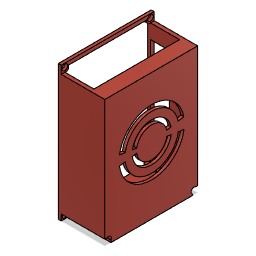
крышка на расбери v2 (Autodesk Fusion 360 design; units mm, degrees)
Autodesk Fusion 360 part; units mm, degrees
sketch "Sketch1" plane through (0, 0, 0) normal (1, 0, 0) x (0, 1, 0)
  line L0 (-75, 50) -> (13, 50)
  line L1 (13, 50) -> (13, -9)
  line L2 (13, -9) -> (-75, -9)
  line L3 (-75, -9) -> (-75, 50)
  circle A0 centre (-75, 50) radius 2
  circle A1 centre (13, 50) radius 2
  circle A2 centre (-75, -9) radius 2
  circle A3 centre (13, -9) radius 2
  line L4 (-77.5, 52.5) -> (-77.5, 47.5)
  line L5 (-77.5, 47.5) -> (-74, 47.5)
  line L6 (-72.5, 49) -> (-72.5, 52.5)
  line L7 (-72.5, 52.5) -> (10, 52.5)
  line L8 (10, 52.5) -> (10, 49)
  line L9 (11.5, 47.5) -> (15.5, 47.5)
  line L10 (15.5, 47.5) -> (15.5, 52.5)
  line L11 (15.5, 52.5) -> (10, 52.5)
  line L12 (-75, 20.5) -> (-35, 20.5)
  line L13 (-77.5, -11.5) -> (-77.5, -6.5)
  line L14 (-77.5, -6.5) -> (-74, -6.5)
  line L15 (-72.5, -8) -> (-72.5, -11.5)
  line L16 (-72.5, -11.5) -> (10, -11.5)
  line L17 (10, -11.5) -> (10, -8)
  line L18 (11.5, -6.5) -> (15.5, -6.5)
  line L19 (15.5, -6.5) -> (15.5, -11.5)
  line L20 (15.5, -11.5) -> (10, -11.5)
  line L21 (-77.5, 52.5) -> (-72.5, 52.5)
  line L22 (-77.5, 47.5) -> (-77.5, -11.5)
  line L23 (-77.5, -11.5) -> (-72.5, -11.5)
  arc A4 (-74, 47.5) -> (-72.5, 49) centre (-74, 49) ccw
  arc A5 (-72.5, -8) -> (-74, -6.5) centre (-74, -8) ccw
  arc A6 (11.5, -6.5) -> (10, -8) centre (11.5, -8) ccw
  arc A7 (10, 49) -> (11.5, 47.5) centre (11.5, 49) ccw
  line L24 (15.5, 47.5) -> (15.5, -6.5)
  dimension "d1" = 88
  dimension "d2" = 59
  dimension "d3" = 4
  dimension "d4" = 4
  dimension "d5" = 4
  dimension "d6" = 4
  dimension "d7" = 1.5
  constraint horizontal L0
  constraint vertical L1
  constraint horizontal L2
  constraint vertical L3
  constraint coincident L0.start L3.end
  constraint coincident L0.end L1.start
  constraint coincident L2.end L3.start
  constraint coincident L1.end L2.start
  constraint perpendicular L0 L4
  constraint perpendicular L4 L5
  constraint perpendicular L0 L6
  constraint perpendicular L3 L7
  constraint perpendicular L7 L8
  constraint perpendicular L8 L9
  constraint perpendicular L9 L10
  constraint perpendicular L8 L11
  constraint midpoint L3 L12.start
  constraint perpendicular L3 L12
  constraint symmetric L4.start L12 L13.start
  constraint symmetric L4.end L12 L13.end
  constraint symmetric L6.end L12 L15.end
  constraint symmetric L7.end L12 L16.end
  constraint symmetric L9.end L12 L18.end
  constraint symmetric L10.end L12 L19.end
  constraint perpendicular L6 L21
  constraint perpendicular L15 L23
  constraint tangent L5 A4
  constraint tangent L6 A4
  constraint tangent L14 A5
  constraint tangent L15 A5
  constraint equal A4 A5
  constraint tangent L17 A6
  constraint tangent L18 A6
  constraint equal A4 A6
  constraint tangent L8 A7
  constraint tangent L9 A7
  constraint equal A4 A7
  constraint perpendicular L18 L24
  measures "d1" distance of L0.start L0.end
  measures "d2" distance of L0.start L2.end
  measures "d3" diameter of A0
  measures "d4" diameter of A1
  measures "d5" diameter of A2
  measures "d6" diameter of A3
  measures "d7" radius of A4
extrude "Extrude1" add sketch "Sketch1" along normal blind 2 contours L0 L3 A0 L4 L5 L6 L21 | L0 L3 A0 L5 L6 A4 | L0 L6 L7 L8 | L3 L5 L14 L22 | L0 L1 A1 L8 L9 L10 L11 | L0 L1 A1 L8 L9 A7 | L2 L3 A2 L14 L15 A5 | L2 L3 A2 L13 L14 L15 L22 L23 | L1 L9 L18 L24 | L2 L15 L16 L17 | L1 L2 A3 L17 L18 L19 L20 | L1 L2 A3 L17 L18 A6
sketch "Sketch2" plane through (2, 0, 0) normal (1, 0, 0) x (0, 1, 0)
  line L0 (-74, -6.5) -> (-75, -6.5)
  line L1 (-75, -6.5) -> (-75, 47.5)
  line L2 (-75, 47.5) -> (-74, 47.5)
  arc A0 (-74, 47.5) -> (-72.5, 49) centre (-74, 49) ccw
  line L3 (-72.5, 49) -> (-72.5, 50)
  line L4 (-72.5, 50) -> (10, 50)
  line L5 (10, 50) -> (10, 49)
  arc A1 (10, 49) -> (11.5, 47.5) centre (11.5, 49) ccw
  line L6 (11.5, 47.5) -> (13, 47.5)
  line L7 (13, 47.5) -> (13, -6.5)
  line L8 (13, -6.5) -> (11.5, -6.5)
  arc A2 (11.5, -6.5) -> (10, -8) centre (11.5, -8) ccw
  line L9 (10, -8) -> (10, -9)
  line L10 (10, -9) -> (-72.5, -9)
  line L11 (-72.5, -9) -> (-72.5, -8)
  arc A3 (-72.5, -8) -> (-74, -6.5) centre (-74, -8) ccw
  circle A4 centre (13, 50) radius 2
  circle A5 centre (13, -9) radius 2
  circle A6 centre (-75, -9) radius 2
  circle A7 centre (-75, 50) radius 2
  line L12 (15.5, 52.5) -> (-77.5, 52.5)
  line L13 (-77.5, 52.5) -> (-77.5, -11.5)
  line L14 (-77.5, -11.5) -> (15.5, -11.5)
  line L15 (15.5, -11.5) -> (15.5, 52.5)
  line L16 (-75.9596, 48.2453) -> (-77.5, 48.2453)
  line L17 (-73.3661, 51.1535) -> (-73.3661, 52.5)
  line L18 (-76.7298, -7.9961) -> (-77.5, -7.9961)
  line L19 (-73.3661, -10.1535) -> (-73.3661, -11.5)
  line L20 (-60.0421, -9) -> (-60.0421, -11.5)
  line L21 (10, 50) -> (10, 52.5)
  line L22 (0, -11.5) -> (0, -9)
  line L23 (10, -9) -> (10, -11.5)
  constraint coincident A7 L16.start
  constraint coincident L13 L16.end
  constraint perpendicular L13 L16
  constraint coincident A7 L17.start
  constraint coincident L12 L17.end
  constraint perpendicular L12 L17
  constraint coincident A6 L18.start
  constraint coincident L13 L18.end
  constraint perpendicular L13 L18
  constraint coincident A6 L19.start
  constraint coincident L14 L19.end
  constraint perpendicular L14 L19
  constraint coincident L10 L20.start
  constraint coincident L14 L20.end
  constraint perpendicular L14 L20
  constraint coincident L4.end L5.start
  constraint coincident L12 L21.end
  constraint perpendicular L12 L21
  constraint coincident L14 L22.start
  constraint coincident L10 L22.end
  constraint perpendicular L10 L22
  constraint coincident L9.end L10.start
  constraint perpendicular L10 L23
extrude "Extrude2" add sketch "Sketch2" along normal blind 30 contours L0 L1 L2 A0 L3 L4 L10 L11 A3 A6 A7 L12 L13 L14 L16 L17 L18 L19 L20 L21 | L10 L14 L22 L23
sketch "Sketch3" plane through (0, 0, 50) normal (0, 0, -1) x (1, 0, 0)
  line L0 (0, 72.5) -> (0, -10)
  line L1 (0, -10) -> (2, -10)
  line L2 (2, -10) -> (32, -10)
  line L3 (32, -10) -> (32, 72.5)
  line L4 (32, 72.5) -> (0, 72.5)
  line L5 (32, -10) -> (18, -10)
  line L6 (18, -10) -> (18, -7.5)
  line L7 (18, -7.5) -> (32, -7.5)
  line L8 (32, -7.5) -> (32, -10)
  dimension "d12" = 14
  dimension "d13" = 2.5
  constraint horizontal L5
  constraint vertical L6
  constraint horizontal L7
  constraint vertical L8
  constraint coincident L2.end L3.start
  measures "d12" distance of L2.end L5.end
  measures "d13" distance of L2.end L7.end
extrude "Extrude3" add sketch "Sketch3" along normal up to surface (59 mm away) contours L2 L3 L5 L6 L7 L8
sketch "Sketch4" plane through (0, 0, 0) normal (0, -1, 0) x (1, 0, 0)
  line L0 (2, -9) -> (2, -11.5)
  line L1 (2, -11.5) -> (32, -11.5)
  line L2 (32, -11.5) -> (32, -9)
  line L3 (32, -9) -> (2, -9)
  line L4 (32, -11.5) -> (15, -11.5)
  line L5 (15, -11.5) -> (15, -9)
  line L6 (15, -9) -> (32, -9)
  line L7 (32, -9) -> (32, -11.5)
  constraint horizontal L4
  constraint vertical L5
  constraint horizontal L6
  constraint vertical L7
  constraint coincident L3 L5.end
  constraint coincident L1.end L2.start
extrude "Extrude4" add sketch "Sketch4" along normal up to surface (60.0421 mm away) contours L1 L2 L3 L4 L5 L6 L7
sketch "Sketch5" plane through (0, 10, 0) normal (0, 1, 0) x (-1, 0, 0)
  line L0 (-2, -11.5) -> (-2, -9)
  line L1 (-2, -9) -> (-18, -9)
  line L2 (-18, -9) -> (-18, 50)
  line L3 (-18, 50) -> (-2, 50)
  line L4 (-2, 50) -> (-2, 52.5)
  line L5 (-2, 52.5) -> (-32, 52.5)
  line L6 (-32, 52.5) -> (-32, -11.5)
  line L7 (-32, -11.5) -> (-2, -11.5)
  line L8 (-18, 29.9805) -> (-22, 29.9805)
  line L9 (-22, 29.9805) -> (-22, -9)
  line L10 (-22, -9) -> (-18, -9)
  constraint coincident L2 L8.start
  constraint perpendicular L2 L8
  constraint perpendicular L1 L9
  constraint coincident L1.end L2.start
  constraint perpendicular L2 L10
extrude "Extrude5" cut sketch "Sketch5" against normal blind 6 contours L2 L8 L9 L10
sketch "Sketch6" plane through (32, 0, 0) normal (1, 0, 0) x (0, 1, 0)
  line L0 (-73.3661, -11.5) -> (10, -11.5)
  line L1 (10, -11.5) -> (10, 52.5)
  line L2 (10, 52.5) -> (-73.3661, 52.5)
  line L3 (-73.3661, 52.5) -> (-73.3661, 51.1535)
  arc A0 (-75.9596, 48.2453) -> (-73.3661, 51.1535) centre (-75, 50) ccw
  line L4 (-75.9596, 48.2453) -> (-77.5, 48.2453)
  line L5 (-77.5, 48.2453) -> (-77.5, -7.9961)
  line L6 (-77.5, -7.9961) -> (-76.7298, -7.9961)
  arc A1 (-73.3661, -10.1535) -> (-76.7298, -7.9961) centre (-75, -9) ccw
  line L7 (-73.3661, -10.1535) -> (-73.3661, -11.5)
  line L8 (7.5, -9) -> (-72.5, -9)
  line L9 (-72.5, -9) -> (-72.5, -8)
  arc A2 (-72.5, -8) -> (-74, -6.5) centre (-74, -8) ccw
  line L10 (-74, -6.5) -> (-75, -6.5)
  line L11 (-75, -6.5) -> (-75, 47.5)
  line L12 (-75, 47.5) -> (-74, 47.5)
  arc A3 (-74, 47.5) -> (-72.5, 49) centre (-74, 49) ccw
  line L13 (-72.5, 49) -> (-72.5, 50)
  line L14 (-72.5, 50) -> (7.5, 50)
  line L15 (7.5, 50) -> (7.5, -9)
  line L16 (-75, 47.5) -> (-73.5326, 47.9393)
  line L17 (-73.5326, 47.9393) -> (-72.7, 50.4)
  line L18 (-72.7, 50.4) -> (9, 51)
  line L19 (9, 51) -> (9, -10.6409)
  line L20 (9, -10.6409) -> (-72.5, -10.6409)
  line L21 (-72.5, -10.6409) -> (-73, -7.5)
  line L22 (-73, -7.5) -> (-74.2896, -6.8066)
  line L23 (-74.2896, -6.8066) -> (-75.5, -6.5)
  line L24 (-75.5, -6.5) -> (-75, 47.5)
  constraint coincident L11.end L12.start
  constraint perpendicular L0 L19
  constraint perpendicular L1 L20
extrude "Extrude6" add sketch "Sketch6" against normal blind 2 contours L8 L9 A2 L10 L11 L12 A3 L13 L14 L15
sketch "Sketch7" plane through (32, 0, 0) normal (1, 0, 0) x (0, 1, 0)
  line L0 (-73.3661, -11.5) -> (10, -11.5)
  line L1 (10, -11.5) -> (10, 52.5)
  line L2 (10, 52.5) -> (-73.3661, 52.5)
  line L3 (-73.3661, 52.5) -> (-73.3661, 51.1535)
  arc A0 (-75.9596, 48.2453) -> (-73.3661, 51.1535) centre (-75, 50) ccw
  line L4 (-75.9596, 48.2453) -> (-77.5, 48.2453)
  line L5 (-77.5, 48.2453) -> (-77.5, -7.9961)
  line L6 (-77.5, -7.9961) -> (-76.7298, -7.9961)
  arc A1 (-73.3661, -10.1535) -> (-76.7298, -7.9961) centre (-75, -9) ccw
  line L7 (-73.3661, -10.1535) -> (-73.3661, -11.5)
  circle A2 centre (-31.6831, 20.1246) radius 22.5
  circle A3 centre (-31.6831, 20.1246) radius 18.5
  circle A4 centre (-31.6831, 20.1246) radius 13.5
  circle A5 centre (-31.6831, 20.1246) radius 10.5
  circle A6 centre (-31.6831, 20.1246) radius 5.7443
  line L8 (-34.7796, 42.4105) -> (-31.6831, 20.1246)
  line L9 (-31.6831, 20.1246) -> (-28.1645, 42.3477)
  line L10 (-31.6831, 20.1246) -> (-35.2016, -2.0986)
  line L11 (-31.6831, 20.1246) -> (-27.4785, -1.9791)
  dimension "d22" = 45
  dimension "d23" = 37
  dimension "d24" = 27
  dimension "d25" = 21
  constraint concentric A2 A3
  constraint concentric A2 A4
  constraint concentric A2 A5
  constraint concentric A3 A6
  constraint coincident A2 L8.start
  constraint coincident A2.centre A3.centre
  constraint coincident A2 L9.end
  constraint coincident A2 L10.end
  constraint parallel L9 L10
  constraint coincident A2 L11.end
  measures "d22" diameter of A2
  measures "d23" diameter of A3
  measures "d24" diameter of A4
  measures "d25" diameter of A5
extrude "Extrude7" cut sketch "Sketch7" against normal blind 4 contours A2 A3 L9 L11 | A2 A3 L8 L10 | A4 A5 L9 L11 | A4 A5 L8 L10
extrude "Extrude8" cut 1 faces at (19.3333, 9.1667, 29.9805) along direction (0, 0, 1) blind 20
